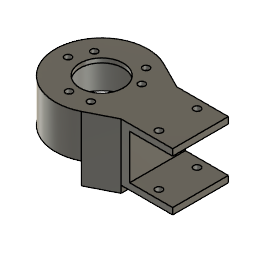
Porta_encoder (Autodesk Fusion 360 design; units mm, degrees)
Autodesk Fusion 360 part; units mm, degrees
note: some values were not read from the file. Set by a fixed rule: which sketch regions a step uses.
sketch "Sketch1" plane through (0, 0, 0) normal (1, 0, 0) x (0, 1, 0)
  line L0 (10, -10.35) -> (-10, -10.35)
  line L1 (-10, -10.35) -> (-10, 10.35)
  line L2 (-10, 10.35) -> (10, 10.35)
  line L3 (10, 10.35) -> (10, -10.35)
  line L4 (10, -10.35) -> (-10, 10.35) construction
  line L5 (-10, -10.35) -> (10, 10.35) construction
  line L6 (12.9717, -13.35) -> (-12.9717, -13.35)
  line L7 (-12.9717, -13.35) -> (-12.9717, 13.35)
  line L8 (-12.9717, 13.35) -> (12.9717, 13.35)
  line L9 (12.9717, 13.35) -> (12.9717, -13.35)
  line L10 (12.9717, -13.35) -> (-12.9717, 13.35) construction
  line L11 (-12.9717, -13.35) -> (12.9717, 13.35) construction
  line L12 (10, 10.35) -> (12.9717, 10.35)
  line L13 (-10, 10.35) -> (-12.9717, 10.35)
  line L14 (-10, -10.35) -> (-12.9717, -10.35)
  line L15 (-12.9717, -10.35) -> (12.9717, -10.35)
  dimension "d1" = 20
  dimension "d2" = 20.7
  dimension "d3" = 26.7
  constraint horizontal L0
  constraint perpendicular L0 L1
  constraint parallel L0 L2
  constraint parallel L1 L3
  constraint coincident L4 origin
  constraint coincident L5 origin
  constraint horizontal L6
  constraint perpendicular L6 L7
  constraint parallel L6 L8
  constraint parallel L7 L9
  constraint coincident L10 origin
  constraint coincident L11 origin
  constraint coincident L9 L12.end
  constraint perpendicular L9 L12
  constraint coincident L7 L13.end
  constraint perpendicular L7 L13
  constraint coincident L7 L14.end
  constraint perpendicular L7 L14
  constraint coincident L9 L15.end
  constraint perpendicular L9 L15
  measures "d1" distance of L1.end L2.end
  measures "d2" distance of L0.end L1.end
  measures "d3" distance of L6.end L7.end
extrude "Extrude1" add sketch "Sketch1" along normal blind 20 contours L0 L6 L7 L9 L14 L15 | L2 L7 L8 L9 L12 L13 makes body 1 at (6.6667, -4.3239, 10.35) makes body 2 at (13.3333, -4.3239, -10.35)
extrude "Extrude2" add sketch "Sketch1" against normal blind 4 separate body contours L0 L1 L2 L3 L15 | L3 L9 L12 L15 | L1 L7 L13 L14 L15 makes body 3
extrude "Extrude3" add sketch "Sketch1" against normal blind 4 contours L0 L6 L7 L9 L14 L15 | L2 L7 L8 L9 L12 L13 bodies 1 2 3
sketch "Sketch2" plane through (0, 0, 13.35) normal (0, 0, 1) x (-1, 0, 0)
  line L0 (4, 12.9717) -> (-20, 12.9717)
  line L1 (-20, 12.9717) -> (-20, -12.9717)
  line L2 (-20, -12.9717) -> (4, -12.9717)
  line L3 (4, -12.9717) -> (4, 12.9717)
  line L4 (4, 0) -> (26, 0)
  circle A0 centre (26, 0) radius 19.55
  circle A1 centre (26, 0) radius 14 construction
  circle A2 centre (26, 0) radius 15.25 construction
  line L5 (26, 0) -> (26, -14)
  circle A3 centre (26, 0) radius 21.5
  line L6 (4, -12.9717) -> (16.3028, -19.1889)
  line L7 (4, 12.9717) -> (16.3028, 19.1889)
  circle A4 centre (26, 0) radius 10.05
  line L8 (-20, -12.9717) -> (-9.5, -12.9717)
  line L9 (-9.5, -12.9717) -> (-9.5, -8.8717)
  circle A5 centre (-9.5, -8.8717) radius 1.6
  line L10 (4, 0) -> (-20, 0) construction
  circle A6 centre (-9.5, 8.8717) radius 1.6
  line L11 (16.3028, -19.1889) -> (16.3028, 19.1889)
  line L12 (26, 0) -> (37.486, -8.0426)
  circle A7 centre (37.486, -8.0426) radius 1.56
  circle A8 centre (27.2221, 13.9685) radius 1.56
  circle A9 centre (13.2919, -5.9259) radius 1.56
  line L13 (26, 0) -> (25.9989, 0)
  line L14 (26, 0) -> (41.25, 0.3993)
  line L15 (26, 0) -> (41, 0) construction
  circle A10 centre (41.25, 0.3993) radius 1.56
  circle A11 centre (18.0292, 13.0072) radius 1.56
  circle A12 centre (18.7208, -13.4066) radius 1.56
  dimension "d22" = 22
  dimension "d23" = 39.1
  dimension "d24" = 28
  dimension "d25" = 30.5
  dimension "d26" = 14
  dimension "d32" = 43
  dimension "d33" = 20.1
  dimension "d38" = 10.5
  dimension "d39" = 4.1
  dimension "d40" = 3.2
  dimension "d56" = 3.12
  dimension "d66" = 1.5
  dimension "d67" = 3.12
  dimension "d68" = 15.25
  dimension "d70" = 360
  constraint midpoint L3 L4.start
  constraint perpendicular L3 L4
  constraint coincident L4.end A0.centre
  constraint concentric A0 A1
  constraint concentric A0 A2
  constraint perpendicular L4 L5
  constraint concentric A2 A3
  constraint coincident L2.end L3.start
  constraint coincident A3 L6.end
  constraint tangent A3 L6
  constraint coincident L0.start L3.end
  constraint coincident A3 L7.end
  constraint tangent A3 L7
  constraint concentric A3 A4
  constraint coincident L1.end L2.start
  constraint coincident L2 L8.end
  constraint parallel L2 L8
  constraint perpendicular L8 L9
  constraint coincident L9.end A5.centre
  constraint midpoint L1 L10.end
  constraint symmetric A5 L10 A6
  constraint coincident L12.end A7.centre
  constraint horizontal L15
  constraint coincident L14.end A10.centre
  measures "d22" distance of L4.start L4.end
  measures "d23" diameter of A0
  measures "d24" diameter of A1
  measures "d25" diameter of A2
  measures "d26" distance of L4.end L5.end
  measures "d32" diameter of A3
  measures "d33" diameter of A4
  measures "d38" distance of L1.end L8.end
  measures "d39" distance of L8.end L9.end
  measures "d40" diameter of A5
  measures "d56" diameter of A7
  measures "d66" angle of L14 L15
  measures "d67" diameter of A10
  measures "d68" horizontal distance of L4.end L14.end
extrude "Extrude4" add sketch "Sketch2" against normal blind 2 separate body contours L4 A0 A4 L11 | A0 A4 L11 | L4 A0 A4 L11 makes body 4
extrude "Extrude5" add sketch "Sketch2" against normal blind 30 contours L3 L4 A3 L7 | L3 L4 A3 L6 | L4 A0 A3 L11 | L4 A0 A3 L11 bodies 1 4
extrude "Extrude6" cut sketch "Sketch2" against normal blind 34 contours A5 | A6 bodies 1
extrude "Extrude7" add sketch "Sketch2" against normal blind 20 contours A0 A3 L11 bodies 1
equation "d68 = ( 30.5 / 2 ) * 1 mm"
